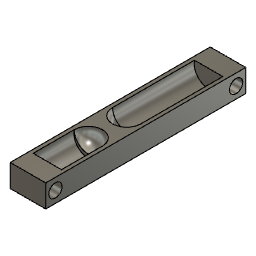
SocketTray (Autodesk Fusion 360 design; units mm, degrees)
Autodesk Fusion 360 part; units mm, degrees
sketch "Sketch1" plane through (0, 0, 0) normal (0, 1, 0) x (1, 0, 0)
  line L0 (0, 0) -> (22, 0)
  line L1 (22, 0) -> (22, -124)
  line L2 (22, -124) -> (0, -124)
  line L3 (0, -124) -> (0, 0)
  dimension "d2" = 124
  dimension "d3" = 22
  constraint horizontal L0
  constraint vertical L1
  constraint horizontal L2
  constraint vertical L3
  constraint coincident L0.start L3.end
  measures "d2" distance of L0.start L2.end
  measures "d3" distance of L0.start L0.end
extrude "Extrude1" add sketch "Sketch1" along normal blind 14
sketch "Sketch2" plane through (0, 0, 124) normal (0, 0, 1) x (1, 0, 0)
  line L0 (0, 0) -> (22, 0)
  line L1 (22, 0) -> (22, 14)
  line L2 (22, 14) -> (0, 14)
  line L3 (0, 14) -> (0, 0)
  circle A0 centre (11, 12) radius 9
  dimension "d10" = 18
  dimension "d30" = 2
  dimension "d31" = 11
  measures "d10" diameter of A0
  measures "d30" distance of L2 A0.centre
  measures "d31" distance of L1 A0.centre
extrude "Extrude2" cut sketch "Sketch2" against normal blind 50.8 from surface at -61.2 contours L2 A0 picked at (10.0242, 9.6203)
sketch "Sketch3" plane through (22, 0, 0) normal (1, 0, 0) x (0, 0, -1)
  line L0 (-124, 0) -> (0, 0)
  line L1 (0, 0) -> (0, 14)
  line L2 (0, 14) -> (-124, 14)
  line L3 (-124, 14) -> (-124, 0)
  circle A0 centre (-6, 7) radius 4.125
  circle A1 centre (-118, 7) radius 4.125
  dimension "d18" = 8.25
  dimension "d21" = 8.25
  dimension "d22" = 7
  dimension "d23" = 6
  dimension "d24" = 7
  dimension "d25" = 6
  measures "d18" diameter of A0
  measures "d21" diameter of A1
  measures "d22" distance of L2 A1.centre
  measures "d23" distance of L3 A1.centre
  measures "d24" distance of L2 A0.centre
  measures "d25" distance of L1 A0.centre
extrude "Extrude3" cut sketch "Sketch3" against normal blind 25 contours A0 | A1
extrude "Extrude5" cut sketch "Sketch2" against normal blind 25.4 from surface at -12 contours L2 A0 picked at (10.0242, 9.6203)
sketch "Sketch10" plane through (0, 14, 0) normal (0, 1, 0) x (-1, 0, 0)
  line L0 (-2.225, 112) -> (-2.225, 86.6)
  line L1 (-2.225, 86.6) -> (-19.775, 86.6)
  line L2 (-19.775, 86.6) -> (-19.775, 112)
  line L3 (-19.775, 112) -> (-2.225, 112)
  line L4 (-2.225, 62.8) -> (-2.225, 12)
  line L5 (-2.225, 12) -> (-19.775, 12)
  line L6 (-19.775, 12) -> (-19.775, 62.8)
  line L7 (-19.775, 62.8) -> (-2.225, 62.8)
  line L8 (0, 124) -> (-22, 124)
  line L9 (-22, 124) -> (-22, 0)
  line L10 (-22, 0) -> (0, 0)
  line L11 (0, 0) -> (0, 124)
  circle A0 centre (-11, 86.6) radius 8.775
  circle A1 centre (-11, 62.8) radius 8.775
  constraint midpoint L1 A0.centre
  constraint coincident L1.end A0
  constraint midpoint L7 A1.centre
  constraint coincident L6.end A1
revolve "Revolve3" cut sketch "Sketch10" angle 90 about axis through (2.225, 14, 86.6) along (-1, 0, 0) contours L1 A0 picked at (-10.3491, 83.7483)
revolve "Revolve4" cut sketch "Sketch10" angle 90 about axis through (19.775, 14, 62.8) along (1, 0, 0) contours L7 A1 picked at (-12.0686, 65.5228)
equation "d2 = BoxLength + 2 * RailBoxDia"
equation "d3 = SocketExtDia + 4 mm"
equation "SocketExtDia = 17.75 mm + 0.25 mm"
equation "d8 = SocketBoxHeight"
equation "d10 = SocketExtDia"
equation "d11 = -d2 + SocketHeight + RailBoxDia"
equation "d12 = -SocketHeight"
equation "SocketHeight = 50 mm + 0.8 mm"
equation "BoxWidth = 25 mm"
equation "BoxLength = 100 mm"
equation "RailBoxDia = 12 mm"
equation "d18 = RailDia"
equation "d19 = -BoxWidth"
equation "d21 = RailDia"
equation "d22 = SocketBoxHeight / 2"
equation "d23 = RailBoxDia / 2"
equation "d24 = SocketBoxHeight / 2"
equation "d25 = RailBoxDia / 2"
equation "RailDia = 8 mm + 0.25 mm"
equation "SocketBoxHeight = 14 mm"
equation "d30 = SocketSnap"
equation "d31 = d3 / 2"
equation "SocketSnap = 2 mm"
equation "Socket2Height = 25 mm + 0.4 mm"
equation "d42 = -RailBoxDia"
equation "d43 = -Socket2Height"
